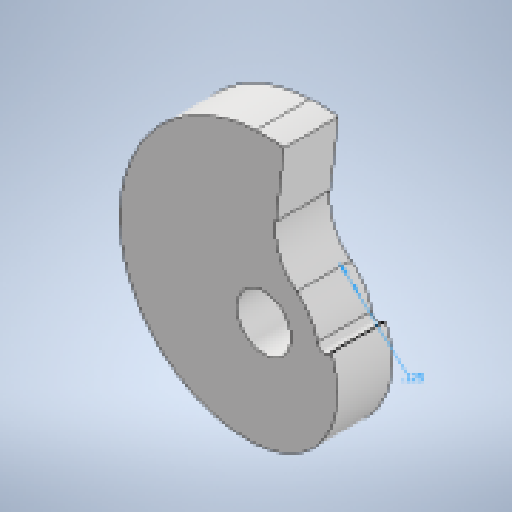
# Autodesk Inventor part: Snail V2
Saved by Autodesk Inventor 2023.2 (Build 272271000, 271)
## iProperties
Created: 2023-11-20
Part Number: Snail V2
Material: UHMW, White
Document SubType Name: Modeling
Designer: Nathan Cai
Density: 0.94 g/cm^3
Appearance: Smooth - White
Author: Nathan Cai
Autodesk Inventor part; units mm, degrees
ref_plane "YZ Plane" through (0, 0, 0) normal (1, 0, 0) x (0, 1, 0)
ref_plane "XZ Plane" through (0, 0, 0) normal (0, 1, 0) x (-1, 0, 0)
ref_plane "XY Plane" through (0, 0, 0) normal (0, 0, 1) x (1, 0, 0)
sketch "Sketch1" plane through (0, 0, 0) normal (0, 0, 1) x (1, 0, 0)
  circle A0 centre (0, 0) radius 3.175
  circle A1 centre (0, 0) radius 19.05
  circle A2 centre (40.4812, 19.05) radius 38.1 construction
  line L0 (2.3815, 18.9005) -> (40.4812, 19.05) construction
  circle A3 centre (0, 0) radius 6.35
  circle A4 centre (0, 0) radius 7.9375 construction
  line L1 (0, 0) -> (2.3815, 18.9005)
  line L2 (0, 0) -> (-0.9367, 19.027) construction
  line L3 (40.4812, 19.05) -> (6.35, 0) construction
  line L4 (0, 0) -> (7.9375, 0) construction
  circle A5 centre (0, 0) radius 12.7 construction
  circle A6 centre (0, 0) radius 16.6688 construction
  arc A7 (0, -12.7) -> (7.8908, 0.86) centre (-1.2714, -2.8843) ccw
  line L5 (0, 0) -> (0, -12.7) construction
  line L6 (0, 0) -> (-19.05, 0) construction
  arc A8 (-16.6688, 0) -> (0, -12.7) centre (-1.914, 2.0767) ccw
  arc A9 (-0.9367, 19.027) -> (-16.6688, 0) centre (-0.1147, 2.33) ccw
  circle A10 centre (7.682, 1.9978) radius 1.5875
  line L7 (7.8908, 0.86) -> (9.2192, 1.6014)
  point P0 (0.7938, 6.3002)
  point P1 (7.2124, 0.4813)
  point P2 (6.1456, 1.5983)
  point P3 (8.0468, 0.4528)
  dimension "d5" = 12.7
  dimension "d15" = 25.4
  dimension "d16" = 33.3375
  dimension "d0" = 6.35
  dimension "d1" = 38.1
  dimension "d2" = 76.2
  dimension "d6" = 15.875
  dimension "d11" = 19.05
  dimension "d12" = 40.4813
  dimension "d13" = 10
  dimension "d14" = 28.943
  dimension "d20" = 3.175
  constraints: 16 end point, 15 point on circle, 8 centre point, 6 coincident, 5 point on line, 3 tangent, 2 horizontal, 1 horizontal alignment, 1 vertical, 1 vertical alignment, 8 other
  measures "d0" diameter of A0
  measures "d1" diameter of A1
  measures "d2" diameter of A2
  measures "d6" diameter of A4
  measures "d11" vertical distance of point (0, 0) L0.end
  measures "d12" horizontal distance of A0.centre L0.end
  measures "d13" angle of L1 L2
  measures "d14" angle of L3 L0
  measures "d20" diameter of A10
extrude "Extrusion1" add sketch "Sketch1" along normal blind 6.35 contours A3 | A3 A10 A7 A8 A9 A1 L1 picked at (-2.1715, 14.5665)
fillet "Fillet1" radius 6.35 1 edges at (0.7938, 6.3002, 3.175)
fillet "Fillet3" radius 0.7937 1 edges at (8.0468, 0.4528, 3.175)
body "Solid1"
